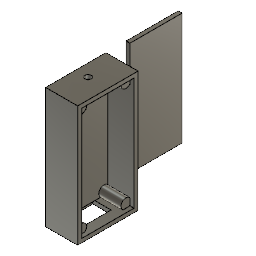
dog_box_v0.1 v0 (Autodesk Fusion 360 design; units mm, degrees)
Autodesk Fusion 360 part; units mm, degrees
note: some values were not read from the file. Set by a fixed rule: which face or edge a step refers to.
sketch "Sketch1" plane through (0, 0, 0) normal (1, 0, 0) x (0, 1, 0)
  line L0 (40, 100) -> (10, 100)
  line L1 (10, 100) -> (10, 40)
  line L2 (10, 40) -> (40, 40)
  line L3 (40, 40) -> (40, 100)
  constraint horizontal L0
  constraint vertical L1
  constraint horizontal L2
  constraint vertical L3
extrude "Extrude1" add sketch "Sketch1" along normal blind 16 thin wall 2 inside makes body 1
sketch "Sketch2" plane through (0, 0, 40) normal (0, 0, -1) x (1, 0, 0)
  line L0 (0, -10) -> (0, -40)
  line L1 (0, -40) -> (16, -40)
  line L2 (16, -40) -> (16, -10)
  line L3 (16, -10) -> (0, -10)
  line L4 (11.0326, -18.5043) -> (2.0224, -18.5043)
  line L5 (2.0224, -18.5043) -> (2.0224, -31.5249)
  line L6 (2.0224, -31.5249) -> (11.0326, -31.5249)
  line L7 (11.0326, -31.5249) -> (11.0326, -18.5043)
  constraint horizontal L4
  constraint vertical L5
  constraint horizontal L6
  constraint vertical L7
extrude "Extrude2" cut sketch "Sketch2" along normal blind 4 and the other way blind 4 contours L4 L5 L6 L7 bodies 1
sketch "Sketch3" plane through (0, 0, 0) normal (-1, 0, 0) x (0, -1, 0)
  line L0 (-12, 42) -> (-38, 42)
  line L1 (-38, 42) -> (-38, 98)
  line L2 (-38, 98) -> (-12, 98)
  line L3 (-12, 98) -> (-12, 42)
  line L4 (-40, 100) -> (-40, 40)
  line L5 (-40, 40) -> (-10, 40)
  line L6 (-10, 40) -> (-10, 100)
  line L7 (-10, 100) -> (-40, 100)
  line L8 (-40, 100) -> (-10, 100)
  line L9 (-10, 100) -> (-10, 40)
  line L10 (-10, 40) -> (-40, 40)
  line L11 (-40, 40) -> (-40, 100)
  constraint horizontal L8
  constraint vertical L9
  constraint horizontal L10
  constraint vertical L11
  constraint coincident L5.end L6.start
  constraint coincident L4.start L7.end
extrude "Extrude3" add sketch "Sketch3" along normal blind 1 and the other way blind 3 contours L0 L1 L2 L3 bodies 1
move_face "MoveFace1" by (1.0202, 0.4525, 0.3793) 1 faces at (-1, 20.6667, 60.6667) on bodies 1
move_face "MoveFace2" by (-0.0311, 0, -0.0882) 1 faces at (0.0202, 20.6667, 60.6667) on bodies 1
cylinder "CylinderPrimitive1" add diameter 4 height 8 placed x (0, 0, -1) y (0, 1, 0) z (1, 0, 0) at (3, 12.5, 42.5) bodies 1
cylinder "CylinderPrimitive2" add diameter 4 height 8 placed x (0, 0, -1) y (0, 1, 0) z (1, 0, 0) at (3, 36.4605, 43.5011) bodies 1
delete_face "DeleteFace1" 2 faces at (8.3333, 34.4605, 43.5024) (8.3333, 37.9075, 42.1205) on bodies 1
delete_face "DeleteFace2" 1 faces at (5.6667, 14.0469, 43.7677) on bodies 1
cylinder "CylinderPrimitive8" add diameter 5 height 11 placed x (0, 0, -1) y (0, 1, 0) z (1, 0, 0) at (3, 14, 44) bodies 1
cylinder "CylinderPrimitive9" add diameter 5 height 11 placed x (0, 0, -1) y (0, 1, 0) z (1, 0, 0) at (3, 36, 44) bodies 1
cylinder "CylinderPrimitive10" add diameter 5 height 11 placed x (0, 0, -1) y (0, 1, 0) z (1, 0, 0) at (3, 14, 96) bodies 1
cylinder "CylinderPrimitive11" add diameter 5 height 11 placed x (0, 0, -1) y (0, 1, 0) z (1, 0, 0) at (3, 36, 96) bodies 1
sketch "Sketch18" plane through (0, 0, 100) normal (0, 0, 1) x (-1, 0, 0)
  line L0 (0, -40) -> (0, -10)
  line L1 (0, -10) -> (-16, -10)
  line L2 (-16, -10) -> (-16, -40)
  line L3 (-16, -40) -> (0, -40)
  circle A0 centre (-6.2053, -25.0092) radius 1.5762
extrude "Extrude4" cut sketch "Sketch18" along normal blind 0 and the other way blind 2 contours A0 bodies 1
sketch "Sketch19" plane through (0, 0, 0) normal (1, 0, 0) x (0, 1, 0)
  line L0 (50, 100) -> (76, 100)
  line L1 (76, 100) -> (76, 44)
  line L2 (76, 44) -> (50, 44)
  line L3 (50, 44) -> (50, 100)
  dimension "d38" = 26
  dimension "d39" = 56
  constraint horizontal L0
  constraint vertical L1
  constraint horizontal L2
  constraint vertical L3
  measures "d38" distance of L0.start L0.end
  measures "d39" distance of L0.start L2.end
extrude "Extrude5" add sketch "Sketch19" along normal blind 2 separate body makes body 2
